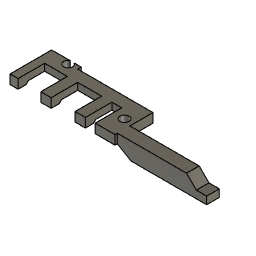
ButtonsAndRC501Holding (Autodesk Fusion 360 design; units mm, degrees)
Autodesk Fusion 360 part; units mm, degrees
sketch "Sketch1" plane through (0, 0, 0) normal (0, 0, 1) x (1, 0, 0)
  line L0 (0, 0) -> (9.1, 0)
  line L1 (9.1, 0) -> (9.1, 17.05)
  line L2 (9.1, 17.05) -> (0, 17.05)
  line L3 (0, 17.05) -> (0, 0)
  line L4 (9.1, 17.05) -> (5, 17.05)
  line L5 (5, 17.05) -> (5, 8.25)
  line L6 (5, 8.25) -> (9.1, 8.25)
  line L7 (9.1, 8.25) -> (9.1, 17.05)
  circle A0 centre (5, 8.25) radius 2
  line L8 (9.1, 0) -> (8.85, 0)
  line L9 (8.85, 0) -> (8.85, 0.25)
  line L10 (8.85, 0.25) -> (9.1, 0.25)
  line L11 (9.1, 0.25) -> (9.1, 0)
  line L12 (0, 17.05) -> (0.25, 17.05)
  line L13 (0.25, 17.05) -> (0.25, 16.8)
  line L14 (0.25, 16.8) -> (0, 16.8)
  line L15 (0, 16.8) -> (0, 17.05)
  line L16 (0.25, 16.8) -> (8.85, 16.8)
  line L17 (8.85, 16.8) -> (8.85, 0.25)
  line L18 (8.85, 0.25) -> (0.25, 0.25)
  line L19 (0.25, 0.25) -> (0.25, 16.8)
  line L20 (0, 0) -> (-5.258, 0)
  line L21 (-5.258, 0) -> (-5.258, 17.05)
  line L22 (-5.258, 17.05) -> (0, 17.05)
  line L23 (0, 17.05) -> (0, 0)
  line L24 (-5.258, 0) -> (-37.05, 0)
  line L25 (-37.05, 0) -> (-37.05, 5)
  line L26 (-37.05, 5) -> (-5.258, 5)
  line L27 (-5.258, 5) -> (-5.258, 0)
  line L28 (-5.258, 0) -> (-37.05, 0)
  line L29 (-37.05, 0) -> (-37.05, 1.5)
  line L30 (-37.05, 1.5) -> (-5.258, 1.5)
  line L31 (-5.258, 1.5) -> (-5.258, 0)
  line L32 (-5.258, 17.05) -> (-10.258, 17.05)
  line L33 (-10.258, 17.05) -> (-10.258, 11.55)
  line L34 (-10.258, 11.55) -> (-5.258, 11.55)
  line L35 (-5.258, 11.55) -> (-5.258, 17.05)
  line L36 (-10.258, 17.05) -> (-18.654, 17.05)
  line L37 (-18.654, 17.05) -> (-18.654, 11.55)
  line L38 (-18.654, 11.55) -> (-10.258, 11.55)
  line L39 (-10.258, 11.55) -> (-10.258, 17.05)
  line L40 (-18.654, 11.55) -> (-23.654, 11.55)
  line L41 (-23.654, 11.55) -> (-23.654, 17.05)
  line L42 (-23.654, 17.05) -> (-18.654, 17.05)
  line L43 (-18.654, 17.05) -> (-18.654, 11.55)
  line L44 (-23.654, 11.55) -> (-42.5, 11.55)
  line L45 (-42.5, 11.55) -> (-42.5, 18.6)
  line L46 (-42.5, 18.6) -> (-23.654, 18.6)
  line L47 (-23.654, 18.6) -> (-23.654, 11.55)
  line L48 (-23.654, 18.6) -> (-18.654, 18.6)
  line L49 (-18.654, 18.6) -> (-18.654, 17.05)
  line L50 (-18.654, 17.05) -> (-23.654, 17.05)
  line L51 (-23.654, 17.05) -> (-23.654, 18.6)
  line L52 (-23.654, 18.6) -> (-27.852, 18.6)
  line L53 (-27.852, 18.6) -> (-27.852, 16.55)
  line L54 (-27.852, 16.55) -> (-23.654, 16.55)
  line L55 (-23.654, 16.55) -> (-23.654, 18.6)
  circle A1 centre (-27.852, 16.55) radius 2
  line L56 (-23.654, 11.55) -> (-18.654, 11.55)
  line L57 (-18.654, 11.55) -> (-18.654, 5)
  line L58 (-18.654, 5) -> (-23.654, 5)
  line L59 (-23.654, 5) -> (-23.654, 11.55)
  line L60 (-5.258, 11.55) -> (-10.258, 11.55)
  line L61 (-10.258, 11.55) -> (-10.258, 5)
  line L62 (-10.258, 5) -> (-5.258, 5)
  line L63 (-5.258, 5) -> (-5.258, 11.55)
  line L64 (-37.05, 5) -> (-32.05, 5)
  line L65 (-32.05, 5) -> (-32.05, 1.5)
  line L66 (-32.05, 1.5) -> (-37.05, 1.5)
  line L67 (-37.05, 1.5) -> (-37.05, 5)
  line L68 (-37.05, 5) -> (-32.05, 5)
  line L69 (-32.05, 5) -> (-32.05, 11.55)
  line L70 (-32.05, 11.55) -> (-37.05, 11.55)
  line L71 (-37.05, 11.55) -> (-37.05, 5)
  line L72 (-23.654, 11.55) -> (-33, 11.55)
  line L73 (-33, 11.55) -> (-37.0503, 15.6003)
  line L74 (-33, 11.55) -> (-27.272, 11.55) construction
  line L75 (-37.0503, 15.6003) -> (-42.5, 15.6003)
  line L76 (-37.0503, 15.6003) -> (-37.05, 11.55)
  line L77 (-37.0503, 15.6003) -> (-37.0503, 18.6)
  line L78 (0, 0) -> (-5.258, 0)
  line L79 (-5.258, 0) -> (-5.258, 5)
  line L80 (-5.258, 5) -> (0, 5)
  line L81 (0, 5) -> (0, 0)
  line L82 (-5.258, 17.05) -> (0, 17.05)
  line L83 (0, 17.05) -> (0, 11.55)
  line L84 (0, 11.55) -> (-5.258, 11.55)
  line L85 (-5.258, 11.55) -> (-5.258, 17.05)
  dimension "d1" = 9.1
  dimension "d2" = 17.05
  dimension "d3" = 4.1
  dimension "d4" = 8.8
  dimension "d5" = 4
  dimension "d6" = 0.25
  dimension "d7" = 0.25
  dimension "d8" = 0.25
  dimension "d9" = 0.25
  dimension "d10" = 5.258
  dimension "d11" = 31.792
  dimension "d12" = 5
  dimension "d13" = 1.5
  dimension "d14" = 5
  dimension "d15" = 5.5
  dimension "d16" = 8.396
  dimension "d17" = 5.5
  dimension "d18" = 5
  dimension "d19" = 5.5
  dimension "d20" = 18.846
  dimension "d21" = 7.05
  dimension "d22" = 4.198
  dimension "d23" = 2.05
  dimension "d24" = 4
  dimension "d25" = 5
  dimension "d26" = 9.346
  dimension "d27" = 135
  dimension "d28" = 5.728
  constraint horizontal L0
  constraint vertical L1
  constraint horizontal L2
  constraint vertical L3
  constraint coincident L0.start L3.end
  constraint horizontal L4
  constraint vertical L5
  constraint horizontal L6
  constraint vertical L7
  constraint coincident L5.end L6.start
  constraint horizontal L8
  constraint vertical L9
  constraint horizontal L10
  constraint vertical L11
  constraint horizontal L12
  constraint vertical L13
  constraint horizontal L14
  constraint vertical L15
  constraint horizontal L16
  constraint vertical L17
  constraint horizontal L18
  constraint vertical L19
  constraint horizontal L20
  constraint vertical L21
  constraint horizontal L22
  constraint vertical L23
  constraint horizontal L24
  constraint vertical L25
  constraint horizontal L26
  constraint vertical L27
  constraint horizontal L28
  constraint vertical L29
  constraint horizontal L30
  constraint vertical L31
  constraint horizontal L32
  constraint vertical L33
  constraint horizontal L34
  constraint vertical L35
  constraint horizontal L36
  constraint vertical L37
  constraint horizontal L38
  constraint vertical L39
  constraint horizontal L40
  constraint vertical L41
  constraint horizontal L42
  constraint vertical L43
  constraint horizontal L44
  constraint vertical L45
  constraint horizontal L46
  constraint vertical L47
  constraint horizontal L48
  constraint vertical L49
  constraint horizontal L50
  constraint vertical L51
  constraint horizontal L52
  constraint vertical L53
  constraint horizontal L54
  constraint vertical L55
  constraint coincident L53.end L54.start
  constraint horizontal L56
  constraint vertical L57
  constraint horizontal L58
  constraint vertical L59
  constraint coincident L26 L57.end
  constraint horizontal L60
  constraint vertical L61
  constraint horizontal L62
  constraint vertical L63
  constraint coincident L26 L61.end
  constraint horizontal L64
  constraint vertical L65
  constraint horizontal L66
  constraint vertical L67
  constraint coincident L30 L65.end
  constraint horizontal L68
  constraint vertical L69
  constraint horizontal L70
  constraint vertical L71
  constraint coincident L44 L69.end
  constraint perpendicular L41 L72
  constraint horizontal L74
  constraint coincident L45 L75.end
  constraint perpendicular L45 L75
  constraint coincident L46 L77.end
  constraint perpendicular L46 L77
  constraint horizontal L78
  constraint vertical L79
  constraint horizontal L80
  constraint vertical L81
  constraint horizontal L82
  constraint vertical L83
  constraint horizontal L84
  constraint vertical L85
  constraint coincident L23 L83.end
  measures "d1" distance of L0.start L0.end
  measures "d2" distance of L0.start L2.end
  measures "d3" distance of L1.end L4.end
  measures "d4" distance of L1.end L6.end
  measures "d5" diameter of A0
  measures "d6" distance of L0.end L8.end
  measures "d7" distance of L0.end L10.end
  measures "d8" distance of L2.end L12.end
  measures "d9" distance of L2.end L14.end
  measures "d10" distance of L0.start L20.end
  measures "d11" distance of L20.end L24.end
  measures "d12" distance of L20.end L26.end
  measures "d13" distance of L20.end L30.end
  measures "d14" distance of L21.end L32.end
  measures "d15" distance of L21.end L34.end
  measures "d16" distance of L32.end L36.end
  measures "d17" distance of L32.end L33.end
  measures "d18" distance of L37.end L40.end
  measures "d19" distance of L37.end L36.end
  measures "d20" distance of L40.end L44.end
  measures "d21" distance of L40.end L46.end
  measures "d22" distance of L46.end L52.end
  measures "d23" distance of L46.end L54.end
  measures "d24" diameter of A1
  measures "d25" distance of L25.end L64.end
  measures "d26" distance of L40.end L72.end
  measures "d27" angle of L73 L74
  measures "d28" distance of L72.end L73.end
extrude "Extrude1" add sketch "Sketch1" along normal blind 2 contours L0 L3 L9 L14 L18 L19 L23 L81 L83 | L3 L20 L21 L23 L27 L31 L78 L79 L80 L81 | L0 L1 L8 L9 L10 L11 | L21 L24 L25 L27 L28 L29 L30 L31 L66 L79 | L1 L6 L10 L17 | L5 L6 A0 L16 L17 L18 L19 | L3 L15 L21 L22 L23 L35 L82 L83 L84 L85 | L21 L26 L34 L60 L61 L62 L63 | L21 L26 L27 L30 L58 L62 L65 L79 | L1 L2 L4 L5 L6 L7 L16 L17 | L5 L6 A0 L16 L17 | L2 L3 L12 L13 L14 L15 L23 L83 | L21 L32 L33 L34 L35 L39 L60 L85 | L25 L26 L30 L64 L65 L66 L67 L68 | L2 L5 L13 L16 | L33 L36 L37 L38 L39 L43 | L26 L40 L56 L57 L58 L59 | L26 L44 L64 L68 L69 L70 L71 L72 | L37 L40 L41 L42 L43 L47 L50 L55 L56 | L41 L44 L46 L47 L53 L54 A1 L70 L72 L73 L77 | L44 L70 L73 L76 | L41 L46 L47 L51 L52 L53 L54 L55 A1 makes body 1
sketch "Sketch2" plane through (0, 0, 2) normal (0, 0, 1) x (-1, 0, 0)
  line L0 (23.654, -5) -> (32.05, -5)
  line L1 (32.05, -5) -> (32.05, -11.55)
  line L2 (32.05, -11.55) -> (23.654, -11.55)
  line L3 (23.654, -11.55) -> (23.654, -5)
  line L4 (18.654, -5) -> (18.654, -11.55)
  line L5 (18.654, -11.55) -> (10.258, -11.55)
  line L6 (10.258, -11.55) -> (10.258, -5)
  line L7 (10.258, -5) -> (18.654, -5)
  line L8 (0, -5) -> (5.258, -5)
  line L9 (5.258, -5) -> (5.258, -11.55)
  line L10 (5.258, -11.55) -> (0, -11.55)
  line L11 (0, -11.55) -> (0, -5)
  circle A0 centre (-5, -8.25) radius 2
  circle A1 centre (27.852, -16.55) radius 2
  line L12 (-9.1, -17.05) -> (23.654, -17.05)
  line L13 (23.654, -17.05) -> (23.654, -18.6)
  line L14 (23.654, -18.6) -> (37.0503, -18.6)
  line L15 (37.0503, -18.6) -> (37.0503, -15.6003)
  line L16 (37.0503, -15.6003) -> (37.05, -11.55)
  line L17 (37.05, -11.55) -> (37.05, 0)
  line L18 (37.05, 0) -> (-9.1, 0)
  line L19 (-9.1, 0) -> (-9.1, -17.05)
  line L20 (32.05, -11.55) -> (32.3, -11.55)
  line L21 (32.3, -11.55) -> (32.3, -11.8)
  line L22 (32.3, -11.8) -> (32.05, -11.8)
  line L23 (32.05, -11.8) -> (32.05, -11.55)
  line L24 (23.654, -5) -> (23.404, -5)
  line L25 (23.404, -5) -> (23.404, -4.75)
  line L26 (23.404, -4.75) -> (23.654, -4.75)
  line L27 (23.654, -4.75) -> (23.654, -5)
  line L28 (18.654, -11.55) -> (18.904, -11.55)
  line L29 (18.904, -11.55) -> (18.904, -11.8)
  line L30 (18.904, -11.8) -> (18.654, -11.8)
  line L31 (18.654, -11.8) -> (18.654, -11.55)
  line L32 (10.258, -5) -> (10.008, -5)
  line L33 (10.008, -5) -> (10.008, -4.75)
  line L34 (10.008, -4.75) -> (10.258, -4.75)
  line L35 (10.258, -4.75) -> (10.258, -5)
  line L36 (5.258, -11.55) -> (5.508, -11.55)
  line L37 (5.508, -11.55) -> (5.508, -11.8)
  line L38 (5.508, -11.8) -> (5.258, -11.8)
  line L39 (5.258, -11.8) -> (5.258, -11.55)
  line L40 (0, -5) -> (-0.25, -5)
  line L41 (-0.25, -5) -> (-0.25, -4.75)
  line L42 (-0.25, -4.75) -> (0, -4.75)
  line L43 (0, -4.75) -> (0, -5)
  line L44 (37.0503, -18.6) -> (36.8003, -18.6)
  line L45 (36.8003, -18.6) -> (36.8003, -18.35)
  line L46 (36.8003, -18.35) -> (37.0503, -18.35)
  line L47 (37.0503, -18.35) -> (37.0503, -18.6)
  line L48 (23.654, -18.6) -> (23.904, -18.6)
  line L49 (23.904, -18.6) -> (23.904, -18.35)
  line L50 (23.904, -18.35) -> (23.654, -18.35)
  line L51 (23.654, -18.35) -> (23.654, -18.6)
  line L52 (37.05, 0) -> (36.8, 0)
  line L53 (36.8, 0) -> (36.8, -0.25)
  line L54 (36.8, -0.25) -> (37.05, -0.25)
  line L55 (37.05, -0.25) -> (37.05, 0)
  line L56 (-9.1, -17.05) -> (-8.85, -17.05)
  line L57 (-8.85, -17.05) -> (-8.85, -16.8)
  line L58 (-8.85, -16.8) -> (-9.1, -16.8)
  line L59 (-9.1, -16.8) -> (-9.1, -17.05)
  line L60 (23.404, -4.75) -> (32.3, -4.75)
  line L61 (32.3, -4.75) -> (32.3, -11.8)
  line L62 (32.3, -11.8) -> (23.404, -11.8)
  line L63 (23.404, -11.8) -> (23.404, -4.75)
  line L64 (18.904, -11.8) -> (10.008, -11.8)
  line L65 (10.008, -11.8) -> (10.008, -4.75)
  line L66 (10.008, -4.75) -> (18.904, -4.75)
  line L67 (18.904, -4.75) -> (18.904, -11.8)
  line L68 (5.508, -11.8) -> (-0.25, -11.8)
  line L69 (-0.25, -11.8) -> (-0.25, -4.75)
  line L70 (-0.25, -4.75) -> (5.508, -4.75)
  line L71 (5.508, -4.75) -> (5.508, -11.8)
  line L72 (-8.85, -16.8) -> (36.8, -16.8)
  line L73 (36.8, -16.8) -> (36.8, -0.25)
  line L74 (36.8, -0.25) -> (-8.85, -0.25)
  line L75 (-8.85, -0.25) -> (-8.85, -16.8)
  line L76 (23.654, -17.05) -> (23.904, -17.05)
  line L77 (23.904, -17.05) -> (23.904, -16.8)
  line L78 (23.904, -16.8) -> (23.654, -16.8)
  line L79 (23.654, -16.8) -> (23.654, -17.05)
  line L80 (23.904, -17.05) -> (36.8003, -17.05)
  line L81 (36.8003, -17.05) -> (36.8003, -18.35)
  line L82 (36.8003, -18.35) -> (23.904, -18.35)
  line L83 (23.904, -18.35) -> (23.904, -17.05)
  line L84 (36.8, -16.8) -> (36.8003, -17.05)
  dimension "d31" = 0.25
  dimension "d32" = 0.25
  dimension "d33" = 0.25
  dimension "d34" = 0.25
  dimension "d35" = 0.25
  dimension "d36" = 0.25
  dimension "d37" = 0.25
  dimension "d38" = 0.25
  dimension "d39" = 0.25
  dimension "d40" = 0.25
  dimension "d41" = 0.25
  dimension "d42" = 0.25
  dimension "d43" = 0.25
  dimension "d44" = 0.25
  dimension "d45" = 0.25
  dimension "d46" = 0.25
  dimension "d47" = 0.25
  dimension "d48" = 0.25
  dimension "d49" = 0.25
  dimension "d50" = 0.25
  dimension "d51" = 0.25
  dimension "d52" = 0.25
  constraint horizontal L20
  constraint vertical L21
  constraint horizontal L22
  constraint vertical L23
  constraint coincident L1.end L2.start
  constraint horizontal L24
  constraint vertical L25
  constraint horizontal L26
  constraint vertical L27
  constraint coincident L0.start L3.end
  constraint horizontal L28
  constraint vertical L29
  constraint horizontal L30
  constraint vertical L31
  constraint coincident L4.end L5.start
  constraint horizontal L32
  constraint vertical L33
  constraint horizontal L34
  constraint vertical L35
  constraint coincident L6.end L7.start
  constraint horizontal L36
  constraint vertical L37
  constraint horizontal L38
  constraint vertical L39
  constraint coincident L9.end L10.start
  constraint horizontal L40
  constraint vertical L41
  constraint horizontal L42
  constraint vertical L43
  constraint coincident L8.start L11.end
  constraint horizontal L44
  constraint vertical L45
  constraint horizontal L46
  constraint vertical L47
  constraint coincident L14.end L15.start
  constraint horizontal L48
  constraint vertical L49
  constraint horizontal L50
  constraint vertical L51
  constraint coincident L13.end L14.start
  constraint horizontal L52
  constraint vertical L53
  constraint horizontal L54
  constraint vertical L55
  constraint coincident L17.end L18.start
  constraint horizontal L56
  constraint vertical L57
  constraint horizontal L58
  constraint vertical L59
  constraint coincident L12.start L19.end
  constraint horizontal L60
  constraint vertical L61
  constraint horizontal L62
  constraint vertical L63
  constraint horizontal L64
  constraint vertical L65
  constraint horizontal L66
  constraint vertical L67
  constraint horizontal L68
  constraint vertical L69
  constraint horizontal L70
  constraint vertical L71
  constraint horizontal L72
  constraint vertical L73
  constraint horizontal L74
  constraint vertical L75
  constraint horizontal L76
  constraint vertical L77
  constraint horizontal L78
  constraint vertical L79
  constraint coincident L12.end L13.start
  constraint horizontal L80
  constraint vertical L81
  constraint horizontal L82
  constraint vertical L83
  measures "d31" distance of L1.end L20.end
  measures "d32" distance of L1.end L22.end
  measures "d33" distance of L0.start L24.end
  measures "d34" distance of L0.start L26.end
  measures "d35" distance of L4.end L28.end
  measures "d36" distance of L4.end L30.end
  measures "d37" distance of L6.end L32.end
  measures "d38" distance of L6.end L34.end
  measures "d39" distance of L9.end L36.end
  measures "d40" distance of L9.end L38.end
  measures "d41" distance of L8.start L40.end
  measures "d42" distance of L8.start L42.end
  measures "d43" distance of L14.end L44.end
  measures "d44" distance of L14.end L46.end
  measures "d45" distance of L13.end L48.end
  measures "d46" distance of L13.end L50.end
  measures "d47" distance of L17.end L52.end
  measures "d48" distance of L17.end L54.end
  measures "d49" distance of L12.start L56.end
  measures "d50" distance of L12.start L58.end
  measures "d51" distance of L12.end L76.end
  measures "d52" distance of L12.end L78.end
extrude "Extrude2" cut sketch "Sketch2" against normal blind 5 contours L0 L1 L20 L27 L60 L61 | L2 L3 L23 L24 L62 L63 | L24 L25 L26 L27 L60 L63 | L20 L21 L22 L23 L61 L62 | L4 L7 L28 L35 L66 L67 | L5 L6 L31 L32 L64 L65 | L28 L29 L30 L31 L64 L67 | L32 L33 L34 L35 L65 L66 | L8 L9 L36 L43 L70 L71 | L10 L11 L39 L40 L68 L69 | L40 L41 L42 L43 L69 L70 | L36 L37 L38 L39 L68 L71 | L72 L76 L77 L78 L79 | L15 L16 L17 L46 L54 L73 L81 L84 | A1 L14 L45 L49 L82 | L13 L50 L76 L83 | L12 L57 L72 L79 | L18 L19 L53 L58 L74 L75 | L17 L18 L52 L53 L54 L55 | L13 L14 L48 L49 L50 L51 | L12 L19 L56 L57 L58 L59 | L14 L15 L44 L45 L46 L47 bodies 1
extrude "Extrude3" add 1 faces at (-5.508, 7.1, 1.3333) along direction (1, 0, 0) blind 1.5 on bodies 1 bodies 1
extrude "Extrude4" cut 1 faces at (-10.008, 9.45, 1.3333) along direction (1, 0, 0) blind 1.5 on bodies 1 bodies 1
extrude "Extrude5" cut 1 faces at (-32.3, 7.1, 1.3333) along direction (-1, 0, 0) blind 1 on bodies 1 bodies 1
sketch "Sketch3" plane through (0, 0, 0) normal (0, 0, -1) x (1, 0, 0)
  line L0 (-33.3, -4.75) -> (-23.404, -4.75)
  line L1 (-23.404, -4.75) -> (-23.404, -11.8)
  line L2 (-23.404, -11.8) -> (-33.3, -11.8)
  line L3 (-33.3, -11.8) -> (-33.3, -4.75)
  line L4 (-8.508, -11.8) -> (-18.904, -11.8)
  line L5 (-18.904, -11.8) -> (-18.904, -4.75)
  line L6 (-18.904, -4.75) -> (-8.508, -4.75)
  line L7 (-8.508, -4.75) -> (-8.508, -11.8)
  line L8 (-26.9802, -18.35) -> (-23.904, -18.35)
  line L9 (-23.904, -18.35) -> (-23.904, -16.8)
  line L10 (-23.904, -16.8) -> (8.85, -16.8)
  line L11 (8.85, -16.8) -> (8.85, -0.25)
  line L12 (8.85, -0.25) -> (-36.8, -0.25)
  line L13 (-36.8, -0.25) -> (-36.8, -16.8)
  line L14 (-36.8, -16.8) -> (-36.8003, -17.05)
  line L15 (-36.8003, -17.05) -> (-36.8003, -18.35)
  line L16 (-36.8003, -18.35) -> (-28.7238, -18.35)
  arc A0 (-26.9802, -18.35) -> (-28.7238, -18.35) centre (-27.852, -16.55) ccw
  circle A1 centre (5, -8.25) radius 2
  line L17 (0.25, -4.75) -> (0.25, -11.8)
  line L18 (0.25, -11.8) -> (-4.008, -11.8)
  line L19 (-4.008, -11.8) -> (-4.008, -4.75)
  line L20 (-4.008, -4.75) -> (0.25, -4.75)
  line L21 (-33.3, -4.75) -> (-36.8, -4.75)
  line L22 (-36.8, -4.75) -> (0.25, -4.75)
  line L23 (0.25, -4.75) -> (0.25, -11.8)
  line L24 (0.25, -11.8) -> (-36.8, -11.8)
  line L25 (-36.8, -11.8) -> (-36.8, -4.75)
  constraint coincident L0.start L3.end
  constraint coincident L13 L21.end
  constraint perpendicular L13 L21
  constraint horizontal L22
  constraint vertical L23
  constraint horizontal L24
  constraint vertical L25
  constraint coincident L17.end L18.start
extrude "Extrude6" cut sketch "Sketch3" against normal blind 1 contours L3 L13 L21 L22 L24 L25 | L1 L5 L22 L24 | L7 L19 L22 L24 bodies 1
chamfer "Chamfer1" distance 1 angle 45 3 edges at (0.25, 8.275, 0) (-18.275, 4.75, 0) (-18.275, 11.8, 0) on bodies 1
sketch "Sketch4" plane through (0, 0, 2) normal (0, 0, 1) x (-1, 0, 0)
  line L0 (23.904, -18.35) -> (26.9802, -18.35)
  arc A0 (28.7238, -18.35) -> (26.9802, -18.35) centre (27.852, -16.55) ccw
  line L1 (28.7238, -18.35) -> (36.8003, -18.35)
  line L2 (36.8003, -18.35) -> (36.8003, -17.05)
  line L3 (36.8003, -17.05) -> (36.8, -16.8)
  line L4 (36.8, -16.8) -> (36.8, -0.25)
  line L5 (36.8, -0.25) -> (-8.85, -0.25)
  line L6 (-8.85, -0.25) -> (-8.85, -16.8)
  line L7 (-8.85, -16.8) -> (23.904, -16.8)
  line L8 (23.904, -16.8) -> (23.904, -18.35)
  line L9 (-0.25, -11.8) -> (-0.25, -4.75)
  line L10 (-0.25, -4.75) -> (4.008, -4.75)
  line L11 (4.008, -4.75) -> (4.008, -11.8)
  line L12 (4.008, -11.8) -> (-0.25, -11.8)
  line L13 (18.904, -11.8) -> (8.508, -11.8)
  line L14 (8.508, -11.8) -> (8.508, -4.75)
  line L15 (8.508, -4.75) -> (18.904, -4.75)
  line L16 (18.904, -4.75) -> (18.904, -11.8)
  line L17 (23.404, -4.75) -> (33.3, -4.75)
  line L18 (33.3, -4.75) -> (33.3, -11.8)
  line L19 (33.3, -11.8) -> (23.404, -11.8)
  line L20 (23.404, -11.8) -> (23.404, -4.75)
  circle A1 centre (-5, -8.25) radius 2
  line L21 (-8.85, -0.25) -> (-1.7501, -0.25)
  line L22 (-1.7501, -0.25) -> (-1.7501, -1)
  line L23 (-1.7501, -1) -> (-8.85, -1)
  line L24 (-8.85, -1) -> (-8.85, -0.25)
  line L25 (-8.85, -1) -> (-3.85, -1)
  line L26 (-3.85, -1) -> (-3.85, -7)
  line L27 (-3.85, -7) -> (-8.85, -7)
  line L28 (-8.85, -7) -> (-8.85, -1)
  line L29 (-8.85, -7) -> (-44.65, -7)
  line L30 (-44.65, -7) -> (-44.65, -1)
  line L31 (-44.65, -1) -> (-8.85, -1)
  line L32 (-8.85, -1) -> (-8.85, -7)
  dimension "d64" = 0.75
  dimension "d65" = 5
  dimension "d66" = 6
  dimension "d67" = 35.8
  dimension "d68" = 6
  constraint horizontal L21
  constraint vertical L22
  constraint horizontal L23
  constraint vertical L24
  constraint coincident L5.end L6.start
  constraint horizontal L25
  constraint vertical L26
  constraint horizontal L27
  constraint vertical L28
  constraint horizontal L29
  constraint vertical L30
  constraint horizontal L31
  constraint vertical L32
  measures "d64" distance of L5.end L23.end
  measures "d65" distance of L23.end L25.end
  measures "d66" distance of L23.end L27.end
  measures "d67" distance of L27.end L29.end
  measures "d68" distance of L27.end L23.end
extrude "Extrude7" add sketch "Sketch4" along normal blind 2 separate body contours L6 L28 L29 L30 L31 L32 makes body 2
extrude "Extrude8" add 1 faces at (-11.3193, 15.1333, 2) along direction (0, 0, 1) blind 2 on bodies 1 bodies 1 2
sketch "Sketch5" plane through (0, 0, 4) normal (0, 0, 1) x (-1, 0, 0)
  circle A0 centre (-5, -8.25) radius 2
  line L0 (23.404, -4.75) -> (33.3, -4.75)
  line L1 (33.3, -4.75) -> (33.3, -11.8)
  line L2 (33.3, -11.8) -> (23.404, -11.8)
  line L3 (23.404, -11.8) -> (23.404, -4.75)
  line L4 (18.904, -11.8) -> (8.508, -11.8)
  line L5 (8.508, -11.8) -> (8.508, -4.75)
  line L6 (8.508, -4.75) -> (18.904, -4.75)
  line L7 (18.904, -4.75) -> (18.904, -11.8)
  line L8 (-0.25, -11.8) -> (-0.25, -4.75)
  line L9 (-0.25, -4.75) -> (4.008, -4.75)
  line L10 (4.008, -4.75) -> (4.008, -11.8)
  line L11 (4.008, -11.8) -> (-0.25, -11.8)
  line L12 (-8.85, -1) -> (-44.65, -1)
  line L13 (-44.65, -1) -> (-44.65, -7)
  line L14 (-44.65, -7) -> (-8.85, -7)
  line L15 (-8.85, -7) -> (-8.85, -16.8)
  line L16 (-8.85, -16.8) -> (23.904, -16.8)
  line L17 (23.904, -16.8) -> (23.904, -18.35)
  line L18 (23.904, -18.35) -> (26.9802, -18.35)
  arc A1 (28.7238, -18.35) -> (26.9802, -18.35) centre (27.852, -16.55) ccw
  line L19 (28.7238, -18.35) -> (36.8003, -18.35)
  line L20 (36.8003, -18.35) -> (36.8003, -17.05)
  line L21 (36.8003, -17.05) -> (36.8, -16.8)
  line L22 (36.8, -16.8) -> (36.8, -0.25)
  line L23 (36.8, -0.25) -> (-8.85, -0.25)
  line L24 (-8.85, -0.25) -> (-8.85, -1)
  line L25 (-44.65, -7) -> (-46.75, -7)
  line L26 (-46.75, -7) -> (-46.75, -1)
  line L27 (-46.75, -1) -> (-44.65, -1)
  line L28 (-44.65, -1) -> (-44.65, -7)
  dimension "d73" = 2.1
  constraint horizontal L25
  constraint vertical L26
  constraint horizontal L27
  constraint vertical L28
  constraint coincident L13.end L14.start
  measures "d73" distance of L13.end L25.end
extrude "Extrude9" add sketch "Sketch5" along normal blind 3 separate body contours L13 L25 L26 L27 L28 makes body 3
sketch "Sketch6" plane through (0, 0, 2) normal (0, 0, -1) x (1, 0, 0)
  line L0 (44.65, -1) -> (8.85, -1)
  line L1 (8.85, -1) -> (8.85, -7)
  line L2 (8.85, -7) -> (44.65, -7)
  line L3 (44.65, -7) -> (44.65, -1)
  line L4 (44.65, -1) -> (42.65, -1)
  line L5 (42.65, -1) -> (42.65, -7)
  line L6 (42.65, -7) -> (44.65, -7)
  line L7 (44.65, -7) -> (44.65, -1)
  dimension "d76" = 2
  constraint horizontal L4
  constraint vertical L5
  constraint horizontal L6
  constraint vertical L7
  constraint coincident L0.start L3.end
  measures "d76" distance of L0.start L4.end
extrude "Extrude10" add sketch "Sketch6" along normal blind 3 contours L0 L2 L3 L4 L5 L6 L7 bodies 1
sketch "Sketch7" plane through (44.65, 0, 0) normal (1, 0, 0) x (0, 1, 0)
  line L0 (7, -1) -> (7, 4)
  line L1 (7, 4) -> (1, 4)
  line L2 (1, 4) -> (1, -1)
  line L3 (1, -1) -> (7, -1)
  line L4 (1, -1) -> (7, -1)
  line L5 (7, -1) -> (7, 2)
  line L6 (7, 2) -> (1, 2)
  line L7 (1, 2) -> (1, -1)
  dimension "d79" = 3
  constraint horizontal L4
  constraint vertical L5
  constraint horizontal L6
  constraint vertical L7
  constraint coincident L2.end L3.start
  measures "d79" distance of L2.end L6.end
extrude "Extrude11" add sketch "Sketch7" along normal blind 3.1 contours L0 L2 L3 L4 L5 L6 L7 bodies 1
extrude "Extrude12" cut 1 faces at (45.6833, 5, 2) along direction (0, 0, -1) blind 0.25 on bodies 1 bodies 1
extrude "Extrude13" cut 1 faces at (44.35, 3, -1) along direction (0, 0, 1) blind 0.25 on bodies 1 bodies 1
extrude "Extrude14" add 1 faces at (44.65, 3, 5) along direction (-1, 0, 0) blind 5 on bodies 3 bodies 3 1
extrude "Extrude15" cut 1 faces at (46.05, 3, 4) along direction (0, 0, 1) blind 0.25 on bodies 3 bodies 3
extrude "Extrude16" cut 1 faces at (44.65, 5, 2.5833) along direction (-1, 0, 0) blind 0.5 on bodies 3 bodies 3
extrude "Extrude17" add 1 faces at (20.1167, 5, 2) along direction (0, 0, -1) blind 2 on bodies 3 bodies 3
extrude "Extrude18" add 1 faces at (44.35, 3, -0.75) along direction (0, 0, -1) blind 2 on bodies 3 bodies 3
extrude "Extrude19" cut 1 faces at (46.55, 3, 1.75) along direction (0, 0, -1) blind 2 on bodies 3 bodies 3
extrude "Extrude20" add 1 faces at (45.0167, 5, 4.25) along direction (0, 0, -1) blind 2 on bodies 3 bodies 3
extrude "Extrude21" cut 1 faces at (39.65, 3, 5) along direction (1, 0, 0) blind 13 on bodies 3 bodies 3
extrude "Extrude22" cut 1 faces at (46.75, 5, 3.4167) along direction (-1, 0, 0) blind 2.6 on bodies 3 bodies 3
extrude "Extrude23" cut 1 faces at (47.75, 5, -1.0833) along direction (-1, 0, 0) blind 3.6 on bodies 3 bodies 3
sketch "Sketch8" plane through (0, 0, 4) normal (0, 0, 1) x (-1, 0, 0)
  line L0 (-0.25, -11.8) -> (-0.25, -4.75)
  line L1 (-0.25, -4.75) -> (4.008, -4.75)
  line L2 (4.008, -4.75) -> (4.008, -11.8)
  line L3 (4.008, -11.8) -> (-0.25, -11.8)
  line L4 (18.904, -11.8) -> (8.508, -11.8)
  line L5 (8.508, -11.8) -> (8.508, -4.75)
  line L6 (8.508, -4.75) -> (18.904, -4.75)
  line L7 (18.904, -4.75) -> (18.904, -11.8)
  line L8 (23.404, -4.75) -> (33.3, -4.75)
  line L9 (33.3, -4.75) -> (33.3, -11.8)
  line L10 (33.3, -11.8) -> (23.404, -11.8)
  line L11 (23.404, -11.8) -> (23.404, -4.75)
  circle A0 centre (-5, -8.25) radius 2
  line L12 (-44.15, -1) -> (-44.15, -7)
  line L13 (-44.15, -7) -> (-8.85, -7)
  line L14 (-8.85, -7) -> (-8.85, -16.8)
  line L15 (-8.85, -16.8) -> (23.904, -16.8)
  line L16 (23.904, -16.8) -> (23.904, -18.35)
  line L17 (23.904, -18.35) -> (26.9802, -18.35)
  arc A1 (28.7238, -18.35) -> (26.9802, -18.35) centre (27.852, -16.55) ccw
  line L18 (28.7238, -18.35) -> (36.8003, -18.35)
  line L19 (36.8003, -18.35) -> (36.8003, -17.05)
  line L20 (36.8003, -17.05) -> (36.8, -16.8)
  line L21 (36.8, -16.8) -> (36.8, -0.25)
  line L22 (36.8, -0.25) -> (-8.85, -0.25)
  line L23 (-8.85, -0.25) -> (-8.85, -1)
  line L24 (-8.85, -1) -> (-44.15, -1)
  line L25 (-8.85, -7) -> (-46.75, -7)
  line L26 (-46.75, -7) -> (-46.75, -1)
  line L27 (-46.75, -1) -> (-8.85, -1)
  line L28 (-8.85, -1) -> (-8.85, -7)
  line L29 (-46.75, -7) -> (-46.25, -7)
  line L30 (-46.25, -7) -> (-46.25, -1)
  line L31 (-46.25, -1) -> (-46.75, -1)
  line L32 (-46.75, -1) -> (-46.75, -7)
  dimension "d106" = 37.9
  dimension "d107" = 6
  dimension "d108" = 0.5
  constraint horizontal L25
  constraint vertical L26
  constraint horizontal L27
  constraint vertical L28
  constraint coincident L13.end L14.start
  constraint horizontal L29
  constraint vertical L30
  constraint horizontal L31
  constraint vertical L32
  measures "d106" distance of L13.end L25.end
  measures "d107" distance of L13.end L23.end
  measures "d108" distance of L25.end L29.end
extrude "Extrude24" add sketch "Sketch8" against normal blind 4 contours L12 L25 L27 L30 bodies 3
extrude "Extrude25" cut 1 faces at (43.15, 3, -2.75) along direction (0, 0, 1) blind 2.75 on bodies 3 bodies 3
sketch "Sketch9" plane through (0, 0, 0) normal (0, 0, -1) x (1, 0, 0)
  line L0 (-36.8, -3.75) -> (1.25, -3.75)
  line L1 (1.25, -3.75) -> (1.25, -12.8)
  line L2 (1.25, -12.8) -> (-36.8, -12.8)
  line L3 (-36.8, -12.8) -> (-36.8, -16.8)
  line L4 (-36.8, -16.8) -> (-36.8003, -17.05)
  line L5 (-36.8003, -17.05) -> (-36.8003, -18.35)
  line L6 (-36.8003, -18.35) -> (-28.7238, -18.35)
  arc A0 (-26.9802, -18.35) -> (-28.7238, -18.35) centre (-27.852, -16.55) ccw
  line L7 (-26.9802, -18.35) -> (-23.904, -18.35)
  line L8 (-23.904, -18.35) -> (-23.904, -16.8)
  line L9 (-23.904, -16.8) -> (8.85, -16.8)
  line L10 (8.85, -16.8) -> (8.85, -7)
  line L11 (8.85, -7) -> (46.25, -7)
  line L12 (46.25, -7) -> (46.25, -1)
  line L13 (46.25, -1) -> (8.85, -1)
  line L14 (8.85, -1) -> (8.85, -0.25)
  line L15 (8.85, -0.25) -> (-36.8, -0.25)
  line L16 (-36.8, -0.25) -> (-36.8, -3.75)
  circle A1 centre (5, -8.25) radius 2
  line L17 (46.25, -1) -> (44.15, -1)
  line L18 (44.15, -1) -> (44.15, -7)
  line L19 (44.15, -7) -> (46.25, -7)
  line L20 (46.25, -7) -> (46.25, -1)
  line L21 (46.25, -7) -> (45.75, -7)
  line L22 (45.75, -7) -> (45.75, -1)
  line L23 (45.75, -1) -> (46.25, -1)
  line L24 (46.25, -1) -> (46.25, -7)
  line L25 (45.75, -1) -> (40.75, -1)
  line L26 (40.75, -1) -> (40.75, -7)
  line L27 (40.75, -7) -> (45.75, -7)
  line L28 (45.75, -7) -> (45.75, -1)
  dimension "d113" = 2.1
  dimension "d114" = 0.5
  dimension "d115" = 5
  constraint horizontal L17
  constraint vertical L18
  constraint horizontal L19
  constraint vertical L20
  constraint coincident L12.end L13.start
  constraint horizontal L21
  constraint vertical L22
  constraint horizontal L23
  constraint vertical L24
  constraint coincident L13 L22.end
  constraint coincident L11.end L12.start
  constraint horizontal L25
  constraint vertical L26
  constraint horizontal L27
  constraint vertical L28
  measures "d113" distance of L12.end L17.end
  measures "d114" distance of L11.end L21.end
  measures "d115" distance of L22.end L25.end
extrude "Extrude26" add sketch "Sketch9" along normal blind 8 contours L11 L13 L18 L25 L26 L27 | L11 L13 L17 L18 L19 L22 L25 L27 L28 bodies 3
sketch "Sketch10" plane through (45.75, 0, 0) normal (1, 0, 0) x (0, 1, 0)
  line L0 (7, 0) -> (1, 0)
  line L1 (1, 0) -> (1, -8)
  line L2 (1, -8) -> (7, -8)
  line L3 (7, -8) -> (7, 0)
  line L4 (1, -8) -> (7, -8)
  line L5 (7, -8) -> (7, -3)
  line L6 (7, -3) -> (1, -3)
  line L7 (1, -3) -> (1, -8)
  dimension "d118" = 5
  constraint horizontal L4
  constraint vertical L5
  constraint horizontal L6
  constraint vertical L7
  constraint coincident L1.end L2.start
  measures "d118" distance of L1.end L6.end
extrude "Extrude27" add sketch "Sketch10" along normal blind 3.6 contours L1 L2 L3 L4 L5 L6 L7 bodies 3
extrude "Extrude28" cut 1 faces at (49.35, 3, -4.6667) along direction (-1, 0, 0) blind 0.5 on bodies 3 bodies 3
extrude "Extrude29" cut 1 faces at (46.7833, 5, -3) along direction (0, 0, -1) blind 0.25 on bodies 3 bodies 3
extrude "Extrude30" cut 1 faces at (43.45, 3, -8) along direction (0, 0, 1) blind 0.25 on bodies 3 bodies 3
extrude "Extrude31" add 1 faces at (40.75, 3, -2.5833) along direction (-1, 0, 0) blind 31.9 on bodies 3 bodies 3
sketch "Sketch11" plane through (0, 1, 0) normal (0, -1, 0) x (1, 0, 0)
  line L0 (8.85, -7.75) -> (48.85, -7.75)
  line L1 (48.85, -7.75) -> (48.85, -3.25)
  line L2 (48.85, -3.25) -> (45.75, -3.25)
  line L3 (45.75, -3.25) -> (45.75, 0)
  line L4 (45.75, 0) -> (46.25, 0)
  line L5 (46.25, 0) -> (46.25, 4)
  line L6 (46.25, 4) -> (8.85, 4)
  line L7 (8.85, 4) -> (8.85, 0)
  line L8 (8.85, 0) -> (8.85, -7.75)
  line L9 (8.85, -7.75) -> (45.75, -7.75)
  line L10 (45.75, -7.75) -> (45.75, 0)
  line L11 (45.75, 0) -> (8.85, 0)
  line L12 (8.85, 0) -> (8.85, -7.75)
  line L13 (8.85, 0) -> (16.6, -7.75)
  line L14 (8.85, 0) -> (19.8102, 0) construction
  dimension "d129" = 45
  constraint horizontal L9
  constraint vertical L10
  constraint horizontal L11
  constraint vertical L12
  constraint coincident L3.end L4.start
  constraint coincident L0.start L8.end
  constraint horizontal L14
  constraint coincident L9 L13.end
  measures "d129" angle of L13 L14
extrude "Extrude32" cut sketch "Sketch11" against normal blind 6 contours L0 L8 L9 L12 L13 bodies 3
sketch "Sketch12" plane through (0, 0, -7.75) normal (0, 0, -1) x (1, 0, 0)
  line L0 (16.6, -1) -> (16.6, -7)
  line L1 (16.6, -7) -> (48.85, -7)
  line L2 (48.85, -7) -> (48.85, -1)
  line L3 (48.85, -1) -> (16.6, -1)
  line L4 (48.85, -7) -> (43.85, -7)
  line L5 (43.85, -7) -> (43.85, -1)
  line L6 (43.85, -1) -> (48.85, -1)
  line L7 (48.85, -1) -> (48.85, -7)
  dimension "d132" = 5
  constraint horizontal L4
  constraint vertical L5
  constraint horizontal L6
  constraint vertical L7
  constraint coincident L1.end L2.start
  measures "d132" distance of L1.end L4.end
extrude "Extrude33" cut sketch "Sketch12" against normal blind 1.5 contours L0 L1 L3 L5 bodies 3
extrude "Extrude34" cut 1 faces at (16.6, 3, -7.25) along direction (-1, 0, 0) blind 18 on bodies 3 bodies 3
chamfer "Chamfer2" distance 1 angle 45 1 edges at (43.85, 4, -7.75) on bodies 3
sketch "Sketch13" plane through (0, 0, 4) normal (0, 0, 1) x (-1, 0, 0)
  line L0 (-0.25, -11.8) -> (-0.25, -4.75)
  line L1 (-0.25, -4.75) -> (4.008, -4.75)
  line L2 (4.008, -4.75) -> (4.008, -11.8)
  line L3 (4.008, -11.8) -> (-0.25, -11.8)
  line L4 (18.904, -11.8) -> (8.508, -11.8)
  line L5 (8.508, -11.8) -> (8.508, -4.75)
  line L6 (8.508, -4.75) -> (18.904, -4.75)
  line L7 (18.904, -4.75) -> (18.904, -11.8)
  line L8 (23.404, -4.75) -> (33.3, -4.75)
  line L9 (33.3, -4.75) -> (33.3, -11.8)
  line L10 (33.3, -11.8) -> (23.404, -11.8)
  line L11 (23.404, -11.8) -> (23.404, -4.75)
  circle A0 centre (-5, -8.25) radius 2
  line L12 (-46.25, -7) -> (-8.85, -7)
  line L13 (-8.85, -7) -> (-8.85, -16.8)
  line L14 (-8.85, -16.8) -> (23.904, -16.8)
  line L15 (23.904, -16.8) -> (23.904, -18.35)
  line L16 (23.904, -18.35) -> (26.9802, -18.35)
  arc A1 (28.7238, -18.35) -> (26.9802, -18.35) centre (27.852, -16.55) ccw
  line L17 (28.7238, -18.35) -> (36.8003, -18.35)
  line L18 (36.8003, -18.35) -> (36.8003, -17.05)
  line L19 (36.8003, -17.05) -> (36.8, -16.8)
  line L20 (36.8, -16.8) -> (36.8, -0.25)
  line L21 (36.8, -0.25) -> (-8.85, -0.25)
  line L22 (-8.85, -0.25) -> (-8.85, -1)
  line L23 (-8.85, -1) -> (-46.25, -1)
  line L24 (-46.25, -1) -> (-46.25, -7)
  line L25 (4.008, -4.75) -> (-0.25, -4.75)
  line L26 (-0.25, -4.75) -> (-0.25, -0.25)
  line L27 (-0.25, -0.25) -> (4.008, -0.25)
  line L28 (4.008, -0.25) -> (4.008, -4.75)
  line L29 (18.904, -4.75) -> (8.508, -4.75)
  line L30 (8.508, -4.75) -> (8.508, -0.25)
  line L31 (8.508, -0.25) -> (18.904, -0.25)
  line L32 (18.904, -0.25) -> (18.904, -4.75)
  line L33 (33.3, -4.75) -> (23.404, -4.75)
  line L34 (23.404, -4.75) -> (23.404, -0.25)
  line L35 (23.404, -0.25) -> (33.3, -0.25)
  line L36 (33.3, -0.25) -> (33.3, -4.75)
  constraint horizontal L25
  constraint vertical L26
  constraint horizontal L27
  constraint vertical L28
  constraint coincident L21 L26.end
  constraint coincident L1.end L2.start
  constraint horizontal L29
  constraint vertical L30
  constraint horizontal L31
  constraint vertical L32
  constraint coincident L21 L30.end
  constraint coincident L6.end L7.start
  constraint horizontal L33
  constraint vertical L34
  constraint horizontal L35
  constraint vertical L36
  constraint coincident L21 L34.end
  constraint coincident L8.end L9.start
extrude "Extrude35" cut sketch "Sketch13" against normal blind 7 contours L1 L21 L25 L26 L27 L28 | L6 L21 L29 L30 L31 L32 | L8 L21 L33 L34 L35 L36 bodies 3
sketch "Sketch14" plane through (0, 1, 0) normal (0, -1, 0) x (1, 0, 0)
  line L0 (43.85, -6.75) -> (44.85, -7.75)
  line L1 (44.85, -7.75) -> (48.85, -7.75)
  line L2 (48.85, -7.75) -> (48.85, -3.25)
  line L3 (48.85, -3.25) -> (45.75, -3.25)
  line L4 (45.75, -3.25) -> (45.75, 0)
  line L5 (45.75, 0) -> (46.25, 0)
  line L6 (46.25, 0) -> (46.25, 4)
  line L7 (46.25, 4) -> (8.85, 4)
  line L8 (8.85, 4) -> (8.85, 0)
  line L9 (8.85, 0) -> (15.1, -6.25)
  line L10 (15.1, -6.25) -> (43.85, -6.25)
  line L11 (43.85, -6.25) -> (43.85, -6.75)
extrude "Extrude36" cut sketch "Sketch14" against normal blind 25 bodies 3
sketch "Sketch15" plane through (0, 0, 4) normal (0, 0, 1) x (-1, 0, 0)
  line L0 (-8.85, -0.25) -> (-8.85, -16.8)
  line L1 (-8.85, -16.8) -> (23.904, -16.8)
  line L2 (23.904, -16.8) -> (23.904, -18.35)
  line L3 (23.904, -18.35) -> (26.9802, -18.35)
  arc A0 (28.7238, -18.35) -> (26.9802, -18.35) centre (27.852, -16.55) ccw
  line L4 (28.7238, -18.35) -> (36.8003, -18.35)
  line L5 (36.8003, -18.35) -> (36.8003, -17.05)
  line L6 (36.8003, -17.05) -> (36.8, -16.8)
  line L7 (36.8, -16.8) -> (36.8, -0.25)
  line L8 (36.8, -0.25) -> (33.3, -0.25)
  line L9 (33.3, -0.25) -> (33.3, -11.8)
  line L10 (33.3, -11.8) -> (23.404, -11.8)
  line L11 (23.404, -11.8) -> (23.404, -0.25)
  line L12 (23.404, -0.25) -> (18.904, -0.25)
  line L13 (18.904, -0.25) -> (18.904, -11.8)
  line L14 (18.904, -11.8) -> (8.508, -11.8)
  line L15 (8.508, -11.8) -> (8.508, -0.25)
  line L16 (8.508, -0.25) -> (4.008, -0.25)
  line L17 (4.008, -0.25) -> (4.008, -11.8)
  line L18 (4.008, -11.8) -> (-0.25, -11.8)
  line L19 (-0.25, -11.8) -> (-0.25, -0.25)
  line L20 (-0.25, -0.25) -> (-8.85, -0.25)
  circle A1 centre (-5, -8.25) radius 2
  line L21 (-8.85, -0.25) -> (-48.25, -0.25)
  line L22 (-48.25, -0.25) -> (-48.25, -14)
  line L23 (-48.25, -14) -> (-8.85, -14)
  line L24 (-8.85, -14) -> (-8.85, -0.25)
  line L25 (-8.85, -0.25) -> (-7.8423, -0.25)
  line L26 (-7.8423, -0.25) -> (-7.8423, -1)
  line L27 (-7.8423, -1) -> (-8.85, -1)
  line L28 (-8.85, -1) -> (-8.85, -0.25)
  line L29 (-8.85, -1) -> (-48.25, -1)
  line L30 (-48.25, -1) -> (-48.25, -7)
  line L31 (-48.25, -7) -> (-8.85, -7)
  line L32 (-8.85, -7) -> (-8.85, -1)
  dimension "d142" = 39.4
  dimension "d143" = 0.75
  dimension "d144" = 6
  constraint horizontal L21
  constraint vertical L22
  constraint horizontal L23
  constraint vertical L24
  constraint coincident L0.start L20.end
  constraint horizontal L25
  constraint vertical L26
  constraint horizontal L27
  constraint vertical L28
  constraint horizontal L29
  constraint vertical L30
  constraint horizontal L31
  constraint vertical L32
  measures "d142" distance of L0.start L21.end
  measures "d143" distance of L0.start L27.end
  measures "d144" distance of L27.end L31.end
extrude "Extrude37" add sketch "Sketch15" along normal blind 0.5 separate body contours L0 L22 L24 L29 L30 L31 L32 makes body 4
extrude "Extrude38" add 1 faces at (35.1167, 3, 4) along direction (0, 0, -1) blind 4 on bodies 4 bodies 4 3
sketch "Sketch16" plane through (0, 0, 0) normal (0, 0, -1) x (1, 0, 0)
  line L0 (0.25, -0.25) -> (0.25, -3.75)
  line L1 (0.25, -3.75) -> (1.25, -3.75)
  line L2 (1.25, -3.75) -> (1.25, -12.8)
  line L3 (1.25, -12.8) -> (-36.8, -12.8)
  line L4 (-36.8, -12.8) -> (-36.8, -16.8)
  line L5 (-36.8, -16.8) -> (-36.8003, -17.05)
  line L6 (-36.8003, -17.05) -> (-36.8003, -18.35)
  line L7 (-36.8003, -18.35) -> (-28.7238, -18.35)
  arc A0 (-26.9802, -18.35) -> (-28.7238, -18.35) centre (-27.852, -16.55) ccw
  line L8 (-26.9802, -18.35) -> (-23.904, -18.35)
  line L9 (-23.904, -18.35) -> (-23.904, -16.8)
  line L10 (-23.904, -16.8) -> (8.85, -16.8)
  line L11 (8.85, -16.8) -> (8.85, -7)
  line L12 (8.85, -7) -> (48.25, -7)
  line L13 (48.25, -7) -> (48.25, -1)
  line L14 (48.25, -1) -> (8.85, -1)
  line L15 (8.85, -1) -> (8.85, -0.25)
  line L16 (8.85, -0.25) -> (0.25, -0.25)
  circle A1 centre (5, -8.25) radius 2
  line L17 (8.85, -1) -> (48.25, -1)
  line L18 (48.25, -1) -> (48.25, -7)
  line L19 (48.25, -7) -> (8.85, -7)
  line L20 (8.85, -7) -> (8.85, -1)
  constraint horizontal L17
  constraint vertical L18
  constraint horizontal L19
  constraint vertical L20
  constraint coincident L12.end L13.start
  constraint coincident L14.end L15.start
extrude "Extrude39" add sketch "Sketch16" along normal blind 5 contours L12 L13 L14 L17 L18 L19 L20 bodies 4
sketch "Sketch17" plane through (0, 1, 0) normal (0, -1, 0) x (1, 0, 0)
  line L0 (48.25, -5) -> (48.25, 4.5)
  line L1 (48.25, 4.5) -> (8.85, 4.5)
  line L2 (8.85, 4.5) -> (8.85, 4)
  line L3 (8.85, 4) -> (8.85, 0)
  line L4 (8.85, 0) -> (8.85, -5)
  line L5 (8.85, -5) -> (48.25, -5)
  line L6 (48.25, -5) -> (43.25, -5)
  line L7 (43.25, -5) -> (43.25, 0)
  line L8 (43.25, 0) -> (48.25, 0)
  line L9 (48.25, 0) -> (48.25, -5)
  line L10 (43.25, 0) -> (38.75, 4.5)
  line L11 (43.25, 0) -> (49.614, 0) construction
  line L12 (8.85, 4) -> (48.25, 4)
  line L13 (43.25, 0) -> (39.25, 4)
  dimension "d151" = 5
  dimension "d152" = 5
  dimension "d153" = 135
  constraint horizontal L6
  constraint vertical L7
  constraint horizontal L8
  constraint vertical L9
  constraint coincident L0.start L5.end
  constraint horizontal L11
  constraint coincident L1 L10.end
  constraint coincident L2.end L3.start
  constraint coincident L0 L12.end
  constraint perpendicular L0 L12
  constraint coincident L10 L13.end
  constraint coincident L12 L13.end
  measures "d151" distance of L0.start L6.end
  measures "d152" distance of L0.start L8.end
  measures "d153" angle of L10 L11
extrude "Extrude40" cut sketch "Sketch17" against normal blind 30.5 contours L0 L8 L10 L12 L13 | L0 L1 L10 L12 | L1 L2 L10 L12 bodies 4
sketch "Sketch18" plane through (0, 1, 0) normal (0, -1, 0) x (1, 0, 0)
  line L0 (48.25, 0) -> (43.25, 0)
  line L1 (43.25, 0) -> (39.25, 4)
  line L2 (39.25, 4) -> (8.85, 4)
  line L3 (8.85, 4) -> (8.85, 0)
  line L4 (8.85, 0) -> (8.85, -5)
  line L5 (8.85, -5) -> (48.25, -5)
  line L6 (48.25, -5) -> (48.25, 0)
  line L7 (48.25, 0) -> (47.75, 0)
  line L8 (47.75, 0) -> (47.75, -5)
  line L9 (47.75, -5) -> (48.25, -5)
  line L10 (48.25, -5) -> (48.25, 0)
  line L11 (48.25, -5) -> (8.85, -5)
  line L12 (8.85, -5) -> (8.85, -3.5)
  line L13 (8.85, -3.5) -> (48.25, -3.5)
  line L14 (48.25, -3.5) -> (48.25, -5)
  line L15 (48.25, 0) -> (43.25, 0)
  line L16 (43.25, 0) -> (43.25, -0.25)
  line L17 (43.25, -0.25) -> (48.25, -0.25)
  line L18 (48.25, -0.25) -> (48.25, 0)
  line L19 (43.25, -0.25) -> (39, 4)
  line L20 (43.25, -0.25) -> (49.2604, -0.25) construction
  dimension "d156" = 0.5
  dimension "d157" = 1.5
  dimension "d158" = 0.25
  dimension "d159" = 135
  constraint horizontal L7
  constraint vertical L8
  constraint horizontal L9
  constraint vertical L10
  constraint coincident L0.start L6.end
  constraint horizontal L11
  constraint vertical L12
  constraint horizontal L13
  constraint vertical L14
  constraint coincident L5.end L6.start
  constraint horizontal L15
  constraint vertical L16
  constraint horizontal L17
  constraint vertical L18
  constraint horizontal L20
  constraint coincident L2 L19.end
  measures "d156" distance of L0.start L7.end
  measures "d157" distance of L5.end L13.end
  measures "d158" distance of L0.start L17.end
  measures "d159" angle of L19 L20
extrude "Extrude41" cut sketch "Sketch18" against normal blind 21 contours L0 L6 L7 L8 L10 L15 L17 L18 | L0 L8 L15 L16 L17 | L6 L8 L10 L13 L17 | L1 L2 L16 L19 | L5 L6 L8 L9 L10 L11 L13 L14 | L4 L5 L8 L11 L12 L13 bodies 4
sketch "Sketch19" plane through (0, 1, 0) normal (0, -1, 0) x (1, 0, 0)
  line L0 (8.85, -3.5) -> (47.75, -3.5)
  line L1 (47.75, -3.5) -> (47.75, -0.25)
  line L2 (47.75, -0.25) -> (43.25, -0.25)
  line L3 (43.25, -0.25) -> (39, 4)
  line L4 (39, 4) -> (8.85, 4)
  line L5 (8.85, 4) -> (8.85, 0)
  line L6 (8.85, 0) -> (8.85, -3.5)
  line L7 (8.85, 0) -> (17.5487, -5.0222)
  line L8 (8.85, 0) -> (18.8944, 0) construction
  dimension "d162" = 30
  constraint horizontal L8
  constraint coincident L5.end L6.start
  measures "d162" angle of L7 L8
extrude "Extrude42" cut sketch "Sketch19" against normal blind 52 contours L0 L6 L7 bodies 4
extrude "Extrude43" cut 1 faces at (20.9207, 1, 1.5) along direction (0, 1, 0) blind 0.25 on bodies 4 bodies 4
extrude "Extrude44" cut 1 faces at (20.9207, 7, 1.5) along direction (0, -1, 0) blind 0.25 on bodies 4 bodies 4
